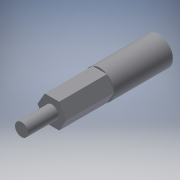
# Autodesk Inventor part: Wheel_Pin
Saved by Autodesk Inventor 2019 (Build 230136000, 136)
## iProperties
Created: 2019-03-02
Part Number: Wheel_Pin
Material: Generic
Document SubType Name: Modeling
Designer: alarr
Density: 1 g/cm^3
Appearance: Default
Author: alarr
Autodesk Inventor part; units mm, degrees
ref_plane "YZ Plane" through (0, 0, 0) normal (1, 0, 0) x (0, 1, 0)
ref_plane "XZ Plane" through (0, 0, 0) normal (0, 1, 0) x (-1, 0, 0)
sketch "Sketch1" plane through (0, 0, 0) normal (0, 0, 1) x (1, 0, 0)
  circle A0 centre (0, 0) radius 4.191 projected
  circle A1 centre (0, 0) radius 4.191
  point P0 (0, 0)
  constraints: 1 centre point, 1 coincident, 1 concentric
ref_plane "Work Plane1" through (-10.4775, -10.4775, 12.7) normal (0, 0, 1) x (1, 0, 0)
extrude "Extrusion1" add sketch "Sketch1" along normal blind 17.145
sketch "Sketch2" plane through (0, 0, 17.145) normal (0, 0, 1) x (1, 0, 0)
  circle A0 centre (0, 0) radius 4.191 projected
  line L0 (-2.0955, -3.6295) -> (-4.191, 0)
  line L1 (-4.191, 0) -> (-2.0955, 3.6295)
  line L2 (-2.0955, 3.6295) -> (2.0955, 3.6295)
  line L3 (2.0955, 3.6295) -> (4.191, 0)
  line L4 (4.191, 0) -> (2.0955, -3.6295)
  line L5 (2.0955, -3.6295) -> (-2.0955, -3.6295)
  point P0 (0, 0)
  point P1 (0, 0)
  constraints: 12 end point, 1 coincident, 1 horizontal, 15 other
extrude "Extrusion2" add sketch "Sketch2" along normal blind 13.97 contours L4 L5 L0 L1 L2 L3
sketch "Sketch3" plane through (0, 0, 31.115) normal (0, 0, 1) x (1, 0, 0)
  circle A0 centre (0, 0) radius 1.905
  dimension "d4" = 3.81
  constraints: 1 centre point, 1 coincident
  measures "d4" diameter of A0
extrude "Extrusion3" add sketch "Sketch3" along normal blind 8.89
body "Solid1"
